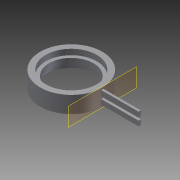
# Autodesk Inventor part: TriggerRing
Saved by Autodesk Inventor 2012 SP2 (Build 160219200, 219)
## iProperties
Created: 2013-07-20
Part Number: TriggerRing
Material: Default
Document SubType Name: Modeling
Designer: 1
Density: 1 g/cm^3
Author: 1
Autodesk Inventor part; units mm, degrees
ref_plane "XZ Plane" through (0, 0, 0) normal (0, 1, 0) x (-1, 0, 0)
sketch "Sketch1" plane through (0, 0, 0) normal (0, 0, 1) x (1, 0, 0)
  line L0 (-34.8016, 76.5) -> (-34.8016, -850)
  line L1 (-34.8016, 76.5) -> (-34.8016, -850)
  line L2 (-14.8016, -585) -> (-14.8016, -580)
  line L3 (-14.8016, -580) -> (-11.8016, -580)
  line L4 (-11.8016, -580) -> (-11.8016, -575)
  line L5 (-11.8016, -575) -> (-6.8016, -575)
  line L6 (-6.8016, -575) -> (-6.8016, -590)
  line L7 (-6.8016, -590) -> (-11.8016, -590)
  line L8 (-11.8016, -590) -> (-11.8016, -585)
  line L9 (-11.8016, -585) -> (-14.8016, -585)
  point P0 (0, 0)
  dimension "d0" = 28
  dimension "d1" = 20
  dimension "d2" = 3
  dimension "d3" = 15
  dimension "d4" = 260
  dimension "d5" = 5
  constraints: 21 end point, 4 parallel, 3 collinear, 3 vertical, 2 perpendicular, 2 other
  measures "d0" distance between parallel lines of L6 L0
  measures "d1" distance between parallel lines of L2 L0
  measures "d2" distance of L2.end L3.end
  measures "d3" distance between parallel lines of L7 L5
  measures "d4" distance from line of L7 L0.end
  measures "d5" distance between parallel lines of L9 L3
revolve "Revolution1" add sketch "Sketch1" angle 360 about axis through (-34.8016, 76.5, 0) along (0, -1, 0)
ref_plane "Work Plane1" through (-6.8016, -582.5, 0) normal (1, 0, 0) x (0, 1, 0)
sketch "Sketch2" plane through (-6.8016, -582.5, 0) normal (1, 0, 0) x (0, 1, 0)
  line L0 (-5.5, 1) -> (-1, 1)
  line L1 (-1, 1) -> (-1, -1)
  line L2 (-1, -1) -> (-5.5, -1)
  line L3 (-5.5, -1) -> (-5.5, 1)
  line L4 (582.5, -1.5) -> (582.5, 1.5) projected
  line L5 (-267.5, 1.5) -> (582.5, 1.5) projected
  line L6 (-267.5, -1.5) -> (-267.5, 1.5) projected
  line L7 (-267.5, -1.5) -> (582.5, -1.5) projected
  line L8 (-7.5, 28) -> (-7.5, -28) projected
  line L9 (1.5, 1) -> (6, 1)
  line L10 (6, 1) -> (6, -1)
  line L11 (6, -1) -> (1.5, -1)
  line L12 (1.5, -1) -> (1.5, 1)
  point P0 (582.5, 0)
  dimension "d7" = 0.5
  dimension "d8" = 0.5
  dimension "d9" = 4.5
  dimension "d10" = 2
  dimension "d13" = 7
  constraints: 16 end point, 2 horizontal, 2 parallel, 1 collinear, 1 perpendicular, 7 other
  measures "d7" distance between parallel lines of L5 L0
  measures "d8" distance between parallel lines of L2 L7
  measures "d9" distance between parallel lines of L1 L3
  measures "d10" distance between parallel lines of L8 L3
  measures "d13" distance of L0.end L10.start
extrude "Extrusion1" add sketch "Sketch2" along normal blind 33.8125 and the other way blind 2.619 contours L0 L1 L2 L3 | L9 L10 L11 L12
ref_plane "Work Plane2" through (-34.8016, -582.5, 28) normal (0, 0, 1) x (1, 0, 0)
sketch "Sketch3" plane through (-34.8016, -582.5, 28) normal (0, 0, 1) x (1, 0, 0)
  circle A0 centre (0, 0) radius 3
  line L0 (27.9821, 6) -> (27.9821, 6) projected
  line L1 (27.9821, 6) -> (27.9821, 1.5) projected
  line L2 (27.9821, 1.5) -> (27.9821, 1.5) projected
  line L3 (27.9821, 1.5) -> (27.9821, 6) projected
  line L4 (27.9821, -1) -> (27.9821, -1) projected
  line L5 (27.9821, -1) -> (27.9821, -5.5) projected
  line L6 (27.9821, -5.5) -> (27.9821, -5.5) projected
  line L7 (27.9821, -5.5) -> (27.9821, -1) projected
  line L8 (-28, -7.5) -> (28, -7.5) projected
  line L9 (-28, 7.5) -> (28, 7.5) projected
  point P0 (34.8016, 582.5)
  dimension "d22" = 6
  dimension "d23" = 7.5
  dimension "d24" = 28
  constraints: 1 centre point
  measures "d22" diameter of A0
  measures "d23" distance from line of L9 A0.centre
  measures "d24" horizontal distance of L9.end A0.centre
extrude "Extrusion2" add sketch "Sketch3" along normal blind 6
body "Solid1"
